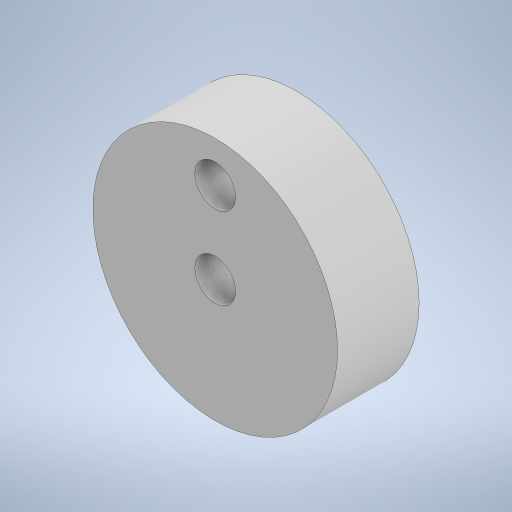
# Autodesk Inventor part: Crank
Saved by Autodesk Inventor 2023 (Build 270158000, 158)
## iProperties
Created: 2022-12-28
Part Number: Crank
Material: Generic
Document SubType Name: Modeling
Designer: tgr41
Density: 1 g/cm^3
Appearance: Default
Author: tgr41
Autodesk Inventor part; units mm, degrees
ref_plane "YZ Plane" through (0, 0, 0) normal (1, 0, 0) x (0, 1, 0)
ref_plane "XZ Plane" through (0, 0, 0) normal (0, 1, 0) x (-1, 0, 0)
ref_plane "XY Plane" through (0, 0, 0) normal (0, 0, 1) x (1, 0, 0)
sketch "Sketch1" plane through (0, 0, 0) normal (0, 0, 1) x (1, 0, 0)
  circle A0 centre (0, 0) radius 19.05
  circle A1 centre (0, 12.7) radius 3.175
  circle A2 centre (0, 0) radius 3.175
  circle A3 centre (0, 0) radius 9.398
  line L0 (0, 0) -> (0, 19.05)
  dimension "d2" = 38.1
  dimension "d3" = 6.35
  dimension "d6" = 6.35
  dimension "d9" = 18.796
  constraints: 3 centre point, 2 end point, 1 coincident, 1 vertical, 1 vertical alignment, 2 other
  measures "d3" diameter of A1
  measures "d6" diameter of A2
  measures "d9" diameter of A3
extrude "Extrusion1" add sketch "Sketch1" along normal blind 12.7 contours A0 | A3
body "Solid1"
